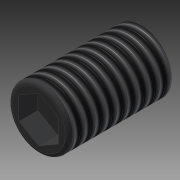
# Autodesk Inventor part: Bolt
Saved by Autodesk Inventor 2014 SP1 (Build 180222100, 222)
## iProperties
Created: 2017-07-09
Part Number: Bolt
Material: Типовые
Document SubType Name: Modeling
Designer: Stepan
Density: 1 g/cm^3
Appearance: Типовые
Author: Stepan
Autodesk Inventor part; units mm, degrees
ref_plane "YZ Plane" through (0, 0, 0) normal (1, 0, 0) x (0, 1, 0)
ref_plane "XZ Plane" through (0, 0, 0) normal (0, 1, 0) x (-1, 0, 0)
ref_plane "XY Plane" through (0, 0, 0) normal (0, 0, 1) x (1, 0, 0)
sketch "Эскиз1" plane through (0, 0, 0) normal (0, 1, 0) x (-1, 0, 0)
  circle A0 centre (0, 0) radius 2
  dimension "d0" = 4
  constraints: 1 centre point, 1 coincident
  measures "d0" diameter of A0
extrude "Выдавливание1" add sketch "Эскиз1" along normal blind 6.75
sketch "Эскиз2" plane through (0, 0, 0) normal (0, -1, 0) x (1, 0, 0)
  circle A0 centre (0, 0) radius 2 projected
  circle A1 centre (0, 0) radius 1.5 construction
  line L0 (0, 1.5) -> (1.299, 0.75)
  line L1 (1.299, 0.75) -> (1.299, -0.75)
  line L2 (1.299, -0.75) -> (0, -1.5)
  line L3 (0, -1.5) -> (-1.299, -0.75)
  line L4 (-1.299, -0.75) -> (-1.299, 0.75)
  line L5 (-1.299, 0.75) -> (0, 1.5)
  dimension "d3" = 3
  constraints: 12 end point, 2 coincident, 1 vertical alignment, 15 other
extrude "Выдавливание2" cut sketch "Эскиз2" against normal blind 1.25 contours L0 L1 L2 L3 L4 L5
fillet "Сопряжение1" radius 0.25 1 edges at (2, 0, 0)
thread "Резьба1" size "M4x0.7" class "6g" standard "ANSI Metric M Profile" full length
